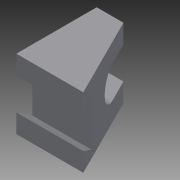
# Autodesk Inventor part: 第一次上机-模型2
Saved by Autodesk Inventor 2013 (Build 170138000, 138)
## iProperties
Created: 2016-11-06
Part Number: 第一次上机-模型2
Material: 常规
Document SubType Name: Modeling
Designer: Administrator
Density: 1 g/cm^3
Author: Administrator
Autodesk Inventor part; units mm, degrees
ref_plane "YZ Plane" through (0, 0, 0) normal (1, 0, 0) x (0, 1, 0)
ref_plane "XZ Plane" through (0, 0, 0) normal (0, 1, 0) x (-1, 0, 0)
ref_plane "XY Plane" through (0, 0, 0) normal (0, 0, 1) x (1, 0, 0)
sketch "草图1" plane through (0, 0, 0) normal (1, 0, 0) x (0, 1, 0)
  line L0 (-30, 0) -> (0, 0)
  line L1 (0, -26) -> (-30, -26)
  line L2 (0, -7) -> (-8, -7)
  arc A0 (-8, -7) -> (-8, -19) centre (-8, -13) ccw
  line L3 (-8, -19) -> (0, -19)
  line L4 (0, 0) -> (0, -7)
  line L5 (0, -19) -> (0, -26)
  line L6 (-30, -7) -> (-24, -3)
  line L7 (-24, -3) -> (-24, -23)
  line L8 (-24, -23) -> (-30, -19)
  line L9 (-8, -13) -> (0, -13) construction
  line L10 (-30, -26) -> (-30, -19)
  line L11 (-30, -7) -> (-30, 0)
  point P0 (-15, 0)
  dimension "d0" = 30
  dimension "d2" = 26
  dimension "d3" = 8
  dimension "d4" = 6
  dimension "d5" = 8
  dimension "d6" = 12
  dimension "d7" = 20
  dimension "d9" = 6
  dimension "d10" = 6
  constraints: 24 end point, 7 parallel, 7 perpendicular, 2 collinear, 2 horizontal alignment, 2 point on circle, 2 tangent, 1 centre point, 1 horizontal, 1 midpoint, 1 vertical alignment, 1 other
  measures "d0" distance of L1.start L1.end
  measures "d2" distance of L1.end L0.start
  measures "d3" distance of L2.start L2.end
  measures "d4" radius of A0
  measures "d5" distance of L9.end L9.start
  measures "d6" distance of L8.end L6.start
  measures "d7" distance of L7.end L6.end
  measures "d9" distance between parallel lines of L10 L7
  measures "d10" distance between parallel lines of L11 L7
extrude "拉伸1" add sketch "草图1" along normal blind 25
sketch "草图2" plane through (0, -30, 0) normal (0, 0, 1) x (1, 0, 0)
  line L0 (0, 0) -> (0, 30) projected
  line L1 (0, 0) -> (25, 0) projected
  line L2 (0, 30) -> (25, 30) projected
  line L3 (25, 0) -> (10, 30)
  dimension "d13" = 10
  constraints: 2 end point, 1 point on line
  measures "d13" distance of L3.end L0.end
extrude "拉伸2" cut sketch "草图2" against normal through all keep common part
